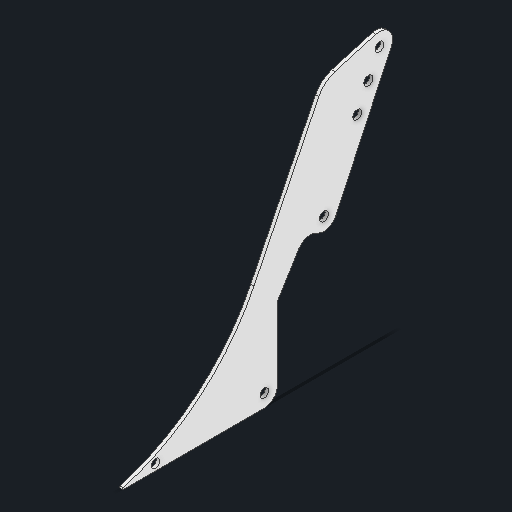
# Autodesk Inventor part: Ramp
Saved by Autodesk Inventor 2025.1 (Build 291241000, 241)
## iProperties
Created: 2024-12-31
Part Number: Ramp
Material: Acetal Resin, White
Document SubType Name: Sheet Metal
Designer: Averey Ku
Density: 1.425 g/cm^3
Appearance: Smooth - White
Flat Pattern Width: 6.5158 cm
Flat Pattern Length: 17.1738 cm
Flat Pattern Area: 111.901 cm^2
Sheet Metal Rule: Default_mm
Sheet Metal Width: 2.565 in
Sheet Metal Length: 6.761 in
Sheet Metal Area: 17.345 in^2
Author: Averey Ku
Autodesk Inventor part; units mm, degrees
ref_plane "YZ Plane" through (0, 0, 0) normal (1, 0, 0) x (0, 1, 0)
ref_plane "XZ Plane" through (0, 0, 0) normal (0, 1, 0) x (-1, 0, 0)
ref_plane "XY Plane" through (0, 0, 0) normal (0, 0, 1) x (1, 0, 0)
sketch "main" plane through (0, 0, 0) normal (0, 0, 1) x (1, 0, 0)
  circle A0 centre (31.5379, -87.1249) radius 2.0955
  circle A1 centre (8.5185, -76.3887) radius 2.0955
  line L0 (52.8956, -28.6403) -> (-10.6273, 2.6327)
  circle A2 centre (1.6034, -31.1233) radius 2.1844
  arc A3 (-63.4783, 65.8273) -> (-10.6273, 2.6327) centre (34.3111, 93.9132) ccw
  line L1 (-57.9066, -8.669) -> (-22.6804, -8.669)
  circle A4 centre (59.152, -57.9639) radius 2.1844
  line L2 (59.4746, -36.466) -> (65.2461, -56.1797)
  arc A5 (63.7627, -62.3301) -> (65.2461, -56.1797) centre (59.152, -57.9639) ccw
  line L3 (-64.2566, 65.7178) -> (-64.2566, -2.319)
  line L4 (-64.2566, 68.6882) -> (6.9552, 68.6882) construction
  arc A6 (-64.2566, -2.319) -> (-57.9066, -8.669) centre (-57.9066, -2.319) ccw
  circle A7 centre (20.0282, -81.7568) radius 2.0955
  arc A8 (28.8539, -92.8798) -> (36.1487, -91.4911) centre (31.5379, -87.1249) ccw
  line L5 (28.8539, -92.8798) -> (5.8344, -82.1435)
  line L6 (36.1487, -91.4911) -> (63.7627, -62.3301)
  circle A9 centre (47.6422, -52.5958) radius 2.2479
  arc A10 (-63.4783, 65.8273) -> (-64.2566, 65.7178) centre (-63.8597, 65.7178) ccw
  arc A11 (59.4746, -36.466) -> (52.8956, -28.6403) centre (47.2862, -40.0344) ccw
  circle A12 centre (36.1325, -47.2277) radius 2.1844
  arc A13 (-3.8107, -27.7809) -> (-4.6861, -32.0859) centre (1.6034, -31.1233) ccw
  line L7 (-3.8107, -27.7809) -> (-3.8107, -27.7809)
  line L8 (-5.8782, -19.0419) -> (-22.6804, -8.669)
  arc A14 (-3.8107, -27.7809) -> (-5.8782, -19.0419) centre (-9.2139, -24.4452) ccw
  circle A15 centre (-61.0816, 50.233) radius 2.0955
  circle A16 centre (-57.9066, -2.319) radius 2.0955
  arc A17 (2.2416, -77.3494) -> (5.8344, -82.1435) centre (8.5185, -76.3887) ccw
  line L9 (2.2416, -77.3494) -> (-4.6861, -32.0859)
  point P0 (22.7298, -27.8341)
  point P1 (-67.4316, 93.9132)
  point P2 (-64.2566, -8.669)
  point P3 (57.9062, -31.1089)
  point P4 (57.9062, -31.1089)
  point P5 (-0.4749, -22.3776)
  point P6 (-1.0693, -36.8975)
  dimension "d4" = 12.7
  dimension "d5" = 4.191
  dimension "d6" = 25.4
  dimension "d10" = 6.35
  dimension "d11" = 4.191
  dimension "d12" = 12.7
  dimension "d14" = 4.4958
  dimension "d23" = 0.3969
  dimension "d25" = 12.7
  dimension "d26" = 12.7
  dimension "d27" = 4.3688
  dimension "d28" = 6.35
  dimension "d29" = 6.35
  dimension "d31" = 4.191
  dimension "d33" = 4.191
  dimension "d35" = 12.7
  dimension "d36" = 12.7
  dimension "d37" = 38.1
  dimension "d38" = 12.7
  measures "d4" diameter of A5
  measures "d5" diameter of A1
  measures "d6" distance of A0.centre A1.centre
  measures "d10" radius of A6
  measures "d11" diameter of A7
  measures "d12" diameter of A8
  measures "d14" diameter of A9
  measures "d23" radius of A10
  measures "d25" distance of A4.centre A9.centre
  measures "d26" radius of A11
  measures "d27" diameter of A12
  measures "d28" distance of L7.start point (-0.475, -22.378)
  measures "d29" radius of A14
  measures "d31" diameter of A15
  measures "d33" diameter of A16
  measures "d35" diameter of A17
  measures "d36" distance of A0.centre point (20.028, -81.757)
  measures "d37" distance of A7.centre A12.centre
  measures "d38" distance of A0.centre A7.centre
sketch "Sketch1" plane through (0, 0, 0) normal (1, 0, 0) x (0, 1, 0)
  circle A0 centre (31.5379, -87.1249) radius 2.0955
  circle A1 centre (8.5185, -76.3887) radius 2.0955
  line L0 (52.8956, -28.6403) -> (-10.6273, 2.6327)
  circle A2 centre (1.6034, -31.1233) radius 2.1844
  arc A3 (-63.4783, 65.8273) -> (-10.6273, 2.6327) centre (34.3111, 93.9132) ccw
  line L1 (-57.9066, -8.669) -> (-22.6804, -8.669)
  circle A4 centre (59.152, -57.9639) radius 2.1844
  line L2 (59.4746, -36.466) -> (65.2461, -56.1797)
  arc A5 (63.7627, -62.3301) -> (65.2461, -56.1797) centre (59.152, -57.9639) ccw
  line L3 (-64.2566, 65.7178) -> (-64.2566, -2.319)
  line L4 (-64.2566, 68.6882) -> (6.9552, 68.6882) construction
  arc A6 (-64.2566, -2.319) -> (-57.9066, -8.669) centre (-57.9066, -2.319) ccw
  circle A7 centre (20.0282, -81.7568) radius 2.0955
  arc A8 (28.8539, -92.8798) -> (36.1487, -91.4911) centre (31.5379, -87.1249) ccw
  line L5 (28.8539, -92.8798) -> (5.8344, -82.1435)
  line L6 (36.1487, -91.4911) -> (63.7627, -62.3301)
  circle A9 centre (47.6422, -52.5958) radius 2.2479
  arc A10 (-63.4783, 65.8273) -> (-64.2566, 65.7178) centre (-63.8597, 65.7178) ccw
  arc A11 (59.4746, -36.466) -> (52.8956, -28.6403) centre (47.2862, -40.0344) ccw
  circle A12 centre (36.1325, -47.2277) radius 2.1844
  arc A13 (-3.8107, -27.7809) -> (-4.6861, -32.0859) centre (1.6034, -31.1233) ccw
  line L7 (-3.8107, -27.7809) -> (-3.8107, -27.7809)
  line L8 (-5.8782, -19.0419) -> (-22.6804, -8.669)
  arc A14 (-3.8107, -27.7809) -> (-5.8782, -19.0419) centre (-9.2139, -24.4452) ccw
  circle A15 centre (-61.0816, 50.233) radius 2.0955
  circle A16 centre (-57.9066, -2.319) radius 2.0955
  arc A17 (2.2416, -77.3494) -> (5.8344, -82.1435) centre (8.5185, -76.3887) ccw
  line L9 (2.2416, -77.3494) -> (-4.6861, -32.0859)
  point P0 (0, 0)
extrude "Extrusion2" add sketch "Sketch1" along normal blind 1.5875
sketch "Sketch2" plane through (1.5875, 0, 0) normal (1, 0, 0) x (0, 0, -1)
  line L0 (82.1435, 5.8344) -> (92.8798, 28.8539) projected
  arc A0 (77.3494, 2.2416) -> (82.1435, 5.8344) centre (76.3887, 8.5185) ccw projected
  line L1 (91.4911, 36.1487) -> (62.3301, 63.7627) projected
  arc A1 (92.8798, 28.8539) -> (91.4911, 36.1487) centre (87.1249, 31.5379) ccw projected
  circle A2 centre (57.9639, 59.152) radius 2.1844 projected
  arc A3 (63.7193, 56.469) -> (62.3301, 63.7627) centre (57.9639, 59.152) ccw
  circle A4 centre (31.1233, 1.6034) radius 2.1844 projected
  arc A5 (32.0859, -4.6861) -> (36.8902, -1.0849) centre (31.1233, 1.6034) ccw
  line L2 (63.7193, 56.469) -> (36.8902, -1.0849)
  line L3 (32.0859, -4.6861) -> (77.3494, 2.2416) projected
  point P0 (0, 0)
  constraints: 4 end point, 4 point on circle, 3 tangent, 2 centre point, 2 coincident
extrude "Extrusion3" cut sketch "Sketch2" against normal blind 25.4 contours A0 L3 A5 L2 A3 L1 A1 L0
equation "\"BendRadius\" = Thickness"
equation "\"BendReliefWidth\" = Thickness"
equation "\"BendReliefDepth\" = 0.5 * Thickness"
equation "\"CornerReliefSize\" = 4 * Thickness"
equation "\"MinimumRemnant\" = 2 * Thickness"
equation "\"TransitionRadius\" = BendRadius"
equation "\"JacobiRadiusSize\" = BendRadius"
equation "\"GapSize\" = Thickness"
equation "\"Thickness\" = 1.5875"
body "Solid2"
